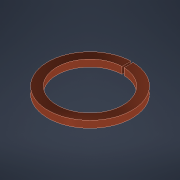
# Autodesk Inventor part: Test_Radiator_Disc
Saved by Autodesk Inventor 2022 (Build 260153000, 153)
## iProperties
Created: 2024-05-10
Part Number: Test_Radiator_Disc
Material: Generic
Document SubType Name: Modeling
Designer: jo_ki
Density: 1 g/cm^3
Appearance: Copper - Polished
Author: jo_ki
Autodesk Inventor part; units mm, degrees
ref_plane "YZ Plane" through (0, 0, 0) normal (1, 0, 0) x (0, 1, 0)
ref_plane "XZ Plane" through (0, 0, 0) normal (0, 1, 0) x (-1, 0, 0)
ref_plane "XY Plane" through (0, 0, 0) normal (0, 0, 1) x (1, 0, 0)
sketch "Sketch1" plane through (0, 0, 0) normal (0, 1, 0) x (-1, 0, 0)
  circle A0 centre (0, 0) radius 20
  circle A1 centre (0, 0) radius 15
  line L0 (-0.5, -14.9917) -> (-0.5, -19.9937)
  line L1 (0.5, -19.9937) -> (0.5, -14.9917)
  line L2 (0, -28) -> (0, 28) projected
  circle A2 centre (0, 0) radius 15.7
  point P0 (-0.5, -15.692)
  point P1 (0.5, -15.692)
  dimension "d0" = 40
  dimension "d1" = 5
  dimension "d2" = 1
  dimension "d5" = 4.3
  constraints: 4 end point, 4 point on circle, 3 centre point, 3 coincident, 1 parallel, 1 vertical, 1 other
  measures "d0" diameter of A0
  measures "d1" radial gap between concentric circles of A0 A1
  measures "d2" distance between parallel lines of L0 L1
  measures "d5" radial gap between concentric circles of A0 A2
extrude "Extrusion1" add sketch "Sketch1" along normal blind 3.25 contours L1 A2 L2 A0 | L2 A2 L0 A0 picked at (18.3995, 1.4835) picked at (-2.823, 18.227)
ref_plane "Work Plane1" through (0, 0, -14.9917) normal (1, 0, 0) x (0, 0, -1)
body "Solid1"
